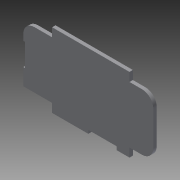
# Autodesk Inventor part: kryt_novy
Saved by Autodesk Inventor 2015 (Build 190159000, 159)
## iProperties
Created: 2015-10-21
Part Number: kryt_novy
Material: Generic
Document SubType Name: Modeling
Designer: Turboslimak
Density: 1 g/cm^3
Appearance: Default
Author: Turboslimak
Autodesk Inventor part; units mm, degrees
ref_plane "YZ Plane" through (0, 0, 0) normal (1, 0, 0) x (0, 1, 0)
ref_plane "XZ Plane" through (0, 0, 0) normal (0, 1, 0) x (-1, 0, 0)
ref_plane "XY Plane" through (0, 0, 0) normal (0, 0, 1) x (1, 0, 0)
sketch "Sketch1" plane through (0, 0, 0) normal (0, 1, 0) x (-1, 0, 0)
  line L0 (-115.003, -50.2) -> (-72.803, -50.2)
  line L1 (-72.803, -50.2) -> (-72.803, -65.6)
  line L2 (-115.003, 50.2) -> (-72.803, 50.2)
  line L3 (-72.803, 50.2) -> (-72.8, 65.6)
  line L4 (-72.803, -50.2) -> (-72.803, -65.6)
  line L5 (-72.8, 50.2) -> (-72.8, 65.6)
  line L6 (-72.8, 65.6) -> (-72.8, 62.6)
  line L7 (114.997, 50.2003) -> (114.9983, 19.2003)
  line L8 (-115.003, -50.2) -> (-115.003, 50.2)
  line L9 (114.997, 50.2003) -> (114.9983, 19.2003)
  line L10 (-72.803, -65.6) -> (-72.803, -50.2)
  line L11 (-72.803, -50.2) -> (-115.003, -50.2)
  line L12 (-115.003, -50.2) -> (-115.003, 50.2)
  line L13 (-115.003, 50.2) -> (-72.8, 50.2)
  line L14 (-72.8, 50.2) -> (-72.8, 65.6)
  line L15 (114.997, 50.2003) -> (63.997, 50.2003)
  line L16 (63.997, 50.2003) -> (63.997, 65.6)
  line L17 (64, -50.1996) -> (64, -65.6)
  line L18 (64, -50.1996) -> (64, -65.6)
  line L19 (-0.003, -65.6) -> (5.997, -65.6) construction
  line L20 (-0.003, -59.6) -> (-50.003, -59.6)
  line L21 (64, -65.6) -> (-0.003, -65.6)
  line L22 (-0.003, -65.6) -> (-0.003, -59.6)
  line L23 (-50.003, -59.6) -> (-50.003, -65.6)
  line L24 (-50.003, -65.6) -> (-72.803, -65.6)
  line L25 (63.997, 65.6) -> (-72.8, 65.6)
  line L26 (114.9983, 19.2003) -> (111.9983, 19.2002)
  line L27 (111.9983, 19.2002) -> (112, -20.8)
  line L28 (64, -50.1996) -> (115, -50.1996)
  line L29 (115, -50.1996) -> (115, -20.8)
  line L30 (115, -20.8) -> (112, -20.8)
  point P0 (0, 0)
  dimension "d0" = 230
  dimension "d2" = 42.2
  dimension "d3" = 15.4
  dimension "d4" = 42.2
  dimension "d5" = 15.4
  dimension "d13" = 31
  dimension "d21" = 6
  dimension "d26" = 3
  dimension "d27" = 51
  dimension "d28" = 51
  constraints: 62 end point, 10 perpendicular, 5 horizontal, 3 collinear, 3 vertical, 1 point on line
  measures "d0" distance of L7.start L2.start
  measures "d2" distance of L0.start L0.end
  measures "d3" distance of L0.end L1.end
  measures "d4" distance of L2.start L2.end
  measures "d5" distance of L2.end L3.end
  measures "d13" distance of L7.start L7.end
  measures "d21" distance of L19.start L20.start
  measures "d26" distance of L7.end L26.end
  measures "d27" distance of L17.start L28.end
  measures "d28" distance of L7.start L15.end
extrude "Extrusion1" add sketch "Sketch1" along normal blind 6 contours L8 L2 L13 L5 L3 L25 L16 L15 L7 L26 L27 L30 L29 L28 L17 L21 L22 L20 L23 L24 L1 L0
fillet "Fillet1" radius 20 3 edges at (115.003, 3, 50.2) (115.003, 3, -50.2) (-114.997, 3, 50.2003)
body "Solid1"
